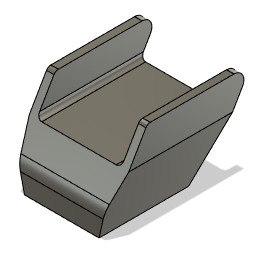
Fimi_Mount (Autodesk Fusion 360 design; units mm, degrees)
Autodesk Fusion 360 part; units mm, degrees
sketch "Skizze2" plane through (0, 0, 0) normal (1, 0, 0) x (0, 0, -1)
  line L0 (0, 0) -> (-36, 0)
  line L1 (0, 0) -> (12.7017, 22)
  line L2 (12.7017, 22) -> (-29.0718, 22)
  line L3 (-29.0718, 22) -> (-36, 10)
  line L4 (-36, 10) -> (-36, 0)
  dimension "d1" = 36
  dimension "d2" = 10
  dimension "d3" = 120
  dimension "d4" = 22
  constraint coincident L0.start L1.start
  constraint horizontal L0
  constraint parallel L0 L2
  constraint perpendicular L0 L4
  constraint parallel L1 L3
  measures "d1" distance of L0.start L0.end
  measures "d2" distance of L0.end L3.end
  measures "d3" angle of L0 L1
  measures "d4" distance of L0 L2
extrude "Extrusion1" add sketch "Skizze2" along normal mid plane 30
sketch "Skizze3" plane through (0, 0, 0) normal (0, -0.5, -0.866025) x (-1, 0, 0)
  line L0 (15, 25.4034) -> (-15, 25.4034)
  line L1 (-15, 25.4034) -> (-15, 0)
  line L2 (-15, 0) -> (15, 0)
  line L3 (15, 0) -> (15, 25.4034)
  line L4 (-15, 25.4034) -> (-17, 25.4034)
  line L5 (-17, 25.4034) -> (-17, 28.021)
  line L6 (-17, 28.021) -> (-17, 40.4034)
  line L7 (-17, 40.4034) -> (-20, 40.4034)
  line L8 (-20, 40.4034) -> (-20, 25.4034)
  line L9 (-20, 25.4034) -> (-15, 0)
  line L10 (-15, 0) -> (-15, 25.4034)
  line L11 (0, 0) -> (0, 25.4034) construction
  line L12 (20, 40.4034) -> (20, 25.4034)
  line L13 (17, 25.4034) -> (17, 28.021)
  line L14 (15, 25.4034) -> (15, 0)
  line L15 (15, 25.4034) -> (17, 25.4034)
  line L16 (20, 25.4034) -> (15, 0)
  line L17 (17, 28.021) -> (17, 40.4034)
  line L18 (17, 40.4034) -> (20, 40.4034)
  line L19 (15, 0) -> (15, 25.4034)
  dimension "d7" = 2
  dimension "d9" = 3
  dimension "d10" = 15
  constraint coincident L0.end L1.start
  constraint perpendicular L1 L4
  constraint perpendicular L4 L5
  constraint perpendicular L4 L6
  constraint perpendicular L6 L7
  constraint perpendicular L7 L8
  constraint coincident L1.end L2.start
  constraint coincident L4 L8.end
  constraint coincident L11.start origin
  constraint midpoint L0 L11.end
  constraint symmetric L0.end L11 L0.start
  constraint symmetric L1.end L11 L2.end
  constraint symmetric L4.end L11 L13.start
  constraint symmetric L5.end L11 L13.end
  constraint symmetric L6.end L11 L17.end
  constraint symmetric L7.end L11 L12.start
  constraint symmetric L8.end L11 L12.end
  measures "d7" distance of L0.end L4.end
  measures "d9" distance of L6.end L7.end
  measures "d10" distance of L4 L7
sweep "Sweeping1" add profiles "Skizze3" along 1 edges at (-15, 22, 8.185) section 1 contours L3 L12 L13 L14 L15 L16 L17 L18 L19 | L1 L4 L5 L6 L7 L8 L9 L10
fillet "Abrundung1" radius 2 2 edges at (-17, 22, 8.185) (17, 22, 8.185)
sketch "Skizze4" plane through (-15, 0, 0) normal (1, 0, 0) x (0, 0, -1)
  line L0 (-36, 0) -> (-36, 10)
  line L1 (-36, 10) -> (-41.7735, 0)
  line L2 (-41.7735, 0) -> (-36, 0)
extrude "Extrusion2" cut sketch "Skizze4" against normal blind 4
extrude "Extrusion3" cut 1 faces at (15, 3.3333, 37.9245) along direction (1, 0, 0) blind 8
fillet "Abrundung2" radius 4 2 edges at (18.5, 34.9904, -20.2017) (-18.5, 34.9904, -20.2017)
fillet "Abrundung3" radius 2 2 edges at (-18.5, 34.9904, 21.5718) (18.5, 34.9904, 21.5718)
fillet "Abrundung4" radius 10 1 edges at (0, 10, 36)
